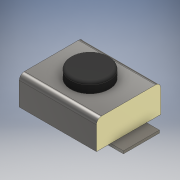
# Autodesk Inventor part: 49-0002
Saved by Autodesk Inventor 2018 (Build 220112000, 112)
## iProperties
Created: 2019-09-25
Part Number: 49-0002
Material: Stainless Steel
Document SubType Name: Modeling
Designer: Bradley
Density: 8 g/cm^3
Appearance: Semi-Polished
Author: Bradley
Autodesk Inventor part; units mm, degrees
ref_plane "YZ Plane" through (0, 0, 0) normal (1, 0, 0) x (0, 1, 0)
ref_plane "XZ Plane" through (0, 0, 0) normal (0, 1, 0) x (-1, 0, 0)
ref_plane "XY Plane" through (0, 0, 0) normal (0, 0, 1) x (1, 0, 0)
sketch "Sketch1" plane through (0, 0, 0) normal (0, 0, 1) x (1, 0, 0)
  line L0 (-1.5, -1.25) -> (1.5, -1.25)
  line L1 (1.5, -1.25) -> (1.5, 1.25)
  line L2 (1.5, 1.25) -> (-1.5, 1.25)
  line L3 (-1.5, 1.25) -> (-1.5, -1.25)
  line L4 (-1.5, -1.25) -> (1.5, 1.25) construction
  line L5 (1.5, -1.25) -> (-1.5, 1.25) construction
  line L6 (-2, 0.7) -> (-1.4, 0.7)
  line L7 (-1.4, 0.7) -> (-1.4, -0.7)
  line L8 (-1.4, -0.7) -> (-2, -0.7)
  line L9 (-2, -0.7) -> (-2, 0.7)
  line L10 (1.4, 0.7) -> (2, 0.7)
  line L11 (2, 0.7) -> (2, -0.7)
  line L12 (2, -0.7) -> (1.4, -0.7)
  line L13 (1.4, -0.7) -> (1.4, 0.7)
  line L14 (0, 1.25) -> (0, -1.25) construction
  point P0 (0, 0)
  point P1 (-2, 0)
  point P2 (0, 0)
  dimension "d0" = 3
  dimension "d1" = 2.5
  dimension "d2" = 4
  dimension "d3" = 1.4
  dimension "d4" = 2.8
  constraints: 30 end point, 6 midpoint, 6 parallel, 3 horizontal, 3 perpendicular, 2 point on line, 1 horizontal alignment, 2 other
  measures "d0" distance of L2.end L1.end
  measures "d1" distance of L1.end L0.end
  measures "d2" distance between parallel lines of L11 L9
  measures "d3" distance of L8.end L6.start
  measures "d4" distance between parallel lines of L13 L7
extrude "Extrusion1" add sketch "Sketch1" along normal blind 1.1 contours L3 L8 L7 L6 L2 L1 L10 L13 L12 L0 | L3 L6 L7 L8 | L12 L13 L10 L1
extrude "Extrusion2" add sketch "Sketch1" against normal blind 0.1 contours L8 L9 L6 L3 | L3 L6 L7 L8 | L12 L13 L10 L1 | L1 L10 L11 L12
sketch "Sketch2" plane through (0, 0, 1.1) normal (0, 0, 1) x (1, 0, 0)
  circle A0 centre (0, 0) radius 0.75
  dimension "d9" = 1.5
  constraints: 1 centre point, 1 coincident
  measures "d9" diameter of A0
extrude "Extrusion3" add sketch "Sketch2" along normal blind 0.4
fillet "Fillet1" radius 0.1 1 edges at (-0.75, 0, 1.5)
fillet "Fillet2" radius 0.2 2 edges at (0, 1.25, 1.1) (0, -1.25, 1.1)
body "Solid1"
